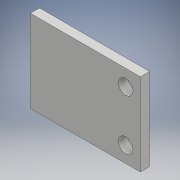
# Autodesk Inventor part: MotorFixer
Saved by Autodesk Inventor 2017 (Build 210142000, 142)
## iProperties
Created: 2016-12-11
Part Number: MotorFixer
Material: Generic
Document SubType Name: Modeling
Designer: umr
Density: 1 g/cm^3
Appearance: Default
Author: umr
Autodesk Inventor part; units mm, degrees
ref_plane "YZ Plane" through (0, 0, 0) normal (1, 0, 0) x (0, 1, 0)
ref_plane "XZ Plane" through (0, 0, 0) normal (0, 1, 0) x (-1, 0, 0)
ref_plane "XY Plane" through (0, 0, 0) normal (0, 0, 1) x (1, 0, 0)
sketch "Sketch1" plane through (0, 0, 0) normal (0, 1, 0) x (-1, 0, 0)
  line L0 (0, 0) -> (60, 0)
  line L1 (60, 0) -> (60, -45)
  line L2 (60, -45) -> (0, -45)
  line L3 (0, -45) -> (0, 0)
  dimension "d0" = 60
  dimension "d1" = 45
  constraints: 8 end point, 2 parallel, 1 horizontal, 1 perpendicular
  measures "d0" distance of L1.end L2.end
  measures "d1" distance of L0.end L1.end
extrude "Extrusion1" add sketch "Sketch1" along normal blind 5
sketch "Sketch2" plane through (0, 5, 0) normal (0, 1, 0) x (1, 0, 0)
  line L0 (-60, 0) -> (0, 0) projected
  line L1 (0, 0) -> (0, 45) projected
  line L2 (0, 45) -> (-60, 45) projected
  line L3 (-60, 45) -> (-60, 0) projected
  circle A0 centre (-8, 36.3) radius 4
  line L4 (-24.9532, 22.5) -> (-60, 22.5)
  circle A1 centre (-8, 8.7) radius 4
  dimension "d5" = 45
  dimension "d7" = 8
  dimension "d8" = 8.7
  dimension "d10" = 8
  constraints: 2 centre point, 2 end point, 1 midpoint, 1 symmetric about line, 1 other
  measures "d5" distance of L0.end L1.end
  measures "d7" diameter of A0
  measures "d8" distance from line of L2 A0.centre
  measures "d10" distance from line of L1 A0.centre
extrude "Extrusion3" cut sketch "Sketch2" against normal up to next contours A0 | A1
equation "\"d7\" = d4"
equation "\"d10\" = d9"
equation "\"d6\" = d4"
equation "\"d9\" = d6"
equation "\"d4\" = 8"
body "Solid1"
